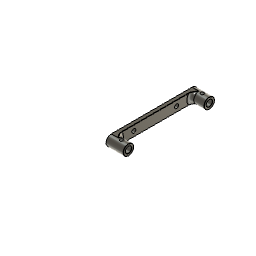
Rail Mount (Autodesk Fusion 360 design; units mm, degrees)
Autodesk Fusion 360 part; units mm, degrees
sketch "Sketch1" plane through (16.4, 0, 0) normal (1, 0, 0) x (0, 1, 0)
  circle A0 centre (3, 27) radius 1.75
  circle A1 centre (87, 27) radius 1.75
  circle A2 centre (15, 13.75) radius 1.75
  circle A3 centre (75, 13.75) radius 1.75
  circle A4 centre (26.5, 5) radius 1.4
  circle A5 centre (63.5, 5) radius 1.4
  line L0 (0, 30) -> (0, 0)
  line L1 (0, 0) -> (90, 0)
  line L2 (90, 0) -> (90, 30)
  line L3 (90, 30) -> (0, 30)
  line L4 (10, 9.1) -> (80, 9.1)
  line L5 (80, 9.1) -> (80, 0)
  line L6 (80, 0) -> (10, 0)
  line L7 (10, 0) -> (10, 9.1)
  line L8 (45, 30) -> (45, 0) construction
  line L9 (10, 4.55) -> (80, 4.55) construction
  circle A6 centre (80, 4.55) radius 2.6
  circle A7 centre (80, 4.55) radius 4.55
  circle A8 centre (10, 4.55) radius 2.6
  circle A9 centre (10, 4.55) radius 4.55
  circle A10 centre (26.5, 4.55) radius 1.75
  circle A11 centre (63.5, 4.55) radius 1.75
  line L10 (14.55, 9.1) -> (14.55, 0)
  line L11 (75.45, 4.55) -> (75.45, 9.1)
  line L12 (75.45, 9.1) -> (75.45, 0)
  point P0 (14.55, 4.55)
  point P1 (75.45, 4.55)
  dimension "d40" = 9.1
  dimension "d41" = 70
  dimension "d42" = 35
  dimension "d43" = 5.2
  dimension "d44" = 9.1
  dimension "d45" = 5.2
  dimension "d46" = 9.1
  dimension "d47" = 3.5
  dimension "d48" = 3.5
  dimension "d49" = 16.5
  dimension "d50" = 37
  dimension "d64" = 9.1
  dimension "d65" = 9.1
  constraint horizontal L4
  constraint vertical L5
  constraint horizontal L6
  constraint vertical L7
  constraint coincident L1 L5.end
  constraint midpoint L3 L8.start
  constraint midpoint L1 L8.end
  constraint midpoint L7 L9.start
  constraint midpoint L5 L9.end
  constraint coincident L9.end A6.centre
  constraint coincident L9.start A8.centre
  constraint coincident L9 A10.centre
  constraint coincident L9 A11.centre
  constraint coincident A9 P0
  constraint coincident L9 P0
  constraint coincident A7 P1
  constraint coincident L9 P1
  constraint vertical L10
  constraint coincident L4 L10.start
  constraint coincident P1 L11.start
  constraint coincident L4 L11.end
  constraint tangent A7 L11
  constraint perpendicular L4 L11
  constraint perpendicular L6 L12
  measures "d40" distance of L4 L6
  measures "d41" distance of L5 L7
  measures "d42" distance of L7 L8
  measures "d43" diameter of A6
  measures "d44" diameter of A7
  measures "d45" diameter of A8
  measures "d46" diameter of A9
  measures "d47" diameter of A10
  measures "d48" diameter of A11
  measures "d49" distance of L7 A10.centre
  measures "d50" distance of A10.centre A11.centre
  measures "d64" distance of L10.start L10.end
  measures "d65" distance of L11.end L12.end
extrude "Extrude1" add sketch "Sketch1" along normal blind 15 contours L7 A8 A9 | L7 A8 A9 | L5 A6 A7 | L5 A6 A7 makes body 1 at (26.4, 14.5274, 5.003) makes body 2 at (26.4, 84.5274, 5.003)
extrude "Extrude2" add sketch "Sketch1" along normal blind 3 contours A4 A10 | A5 A11 | L1 L6 A9 L10 | L1 L4 L6 L10 L11 L12 | L7 A8 | L7 A8 | L4 A9 L10 | L1 L6 A7 L12 | L5 A6 | L5 A6 | L4 A7 L11 L12 picked at (26.6192, 6.3257) picked at (63.6192, 6.3257) bodies 1 2
sketch "Sketch2" plane through (0, 0, 9.1) normal (0, 0, 1) x (-1, 0, 0)
  line L0 (-16.4, -80) -> (-16.4, -10)
  line L1 (-16.4, -10) -> (-19.4, -10)
  line L2 (-19.4, -10) -> (-19.4, -80)
  line L3 (-19.4, -80) -> (-16.4, -80)
  line L4 (-16.4, -10) -> (-31.4, -10) construction
  line L5 (-16.4, -80) -> (-31.4, -80) construction
  line L6 (-25.4, -5) -> (-25.4, -85) construction
  line L7 (-31.4, -5.45) -> (-31.4, -14.55) construction
  circle A0 centre (-25.4, -10) radius 1.4
  circle A1 centre (-25.4, -80) radius 1.4
  dimension "d55" = 6
  dimension "d56" = 2.8
  dimension "d57" = 2.8
  constraint coincident L0.end L1.start
  constraint perpendicular L0 L4
  constraint coincident L0.start L3.end
  constraint perpendicular L2 L5
  constraint perpendicular L5 L6
  constraint coincident L6 A0.centre
  constraint coincident L4 A0.centre
  constraint coincident L5 A1.centre
  constraint coincident L6 A1.centre
  measures "d55" distance of L6 L7
  measures "d56" diameter of A0
  measures "d57" diameter of A1
extrude "Extrude3" cut sketch "Sketch2" against normal blind 4.55 contours A0 | A1 bodies 1
move_body "Move1" bodies 1 to x (1, 0, 0) y (0, 1, 0) z (0, 0, 1) at (0, 0.6116, -13.7601)
fillet "Fillet1" radius 3 2 edges at (19.4, 15.1616, -9.2101) (19.4, 76.0616, -9.2101) on bodies 1
chamfer "Chamfer1" distance 0.2 angle 45 10 edges at (19.4, 45.6116, -4.6601) (20.3687, 77.8102, -4.6601) (20.3687, 13.4129, -4.6601) (19.4, 45.6116, -13.7601) (20.3687, 13.4129, -13.7601) (20.3687, 77.8102, -13.7601) (31.4, 8.1875, -8.2699) (31.4, 6.3695, -10.8555) (31.4, 78.1875, -8.2699) (31.4, 76.3695, -10.8555) on bodies 1
equation "d42 = d41 / 2"
